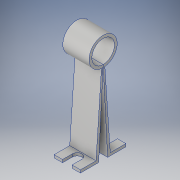
# Autodesk Inventor part: baringstand
Saved by Autodesk Inventor 2018 (Build 220112000, 112)
## iProperties
Created: 2018-02-15
Part Number: baringstand
Material: Aluminum 6061
Document SubType Name: Modeling
Designer: 238438
Density: 2.7 g/cm^3
Appearance: Aluminum - Flat
Author: 238438
Autodesk Inventor part; units mm, degrees
ref_plane "YZ Plane" through (0, 0, 0) normal (1, 0, 0) x (0, 1, 0)
ref_plane "XZ Plane" through (0, 0, 0) normal (0, 1, 0) x (-1, 0, 0)
ref_plane "XY Plane" through (0, 0, 0) normal (0, 0, 1) x (1, 0, 0)
sketch "Sketch2" plane through (0, 0, 0) normal (1, 0, 0) x (0, 1, 0)
  arc A0 (-4.8535, -0.5919) -> (-4.8535, 0.5919) centre (0, 0) ccw
  circle A1 centre (0, 0) radius 3.937
  line L0 (-32.6965, -1.5621) -> (-32.6965, -4.1021)
  line L1 (-31.7186, 2.4716) -> (-4.8535, 0.5919)
  line L2 (-31.7186, -2.4716) -> (-4.8535, -0.5919)
  line L3 (-32.6965, 1.5621) -> (-4.7217, 0.0432)
  line L4 (-32.6965, -1.5621) -> (-4.7217, -0.0423)
  line L5 (-4.7217, 0.0432) -> (-3.937, 0.0003)
  line L6 (-4.7217, -0.0423) -> (-3.937, 0.0003)
  line L7 (-31.7186, -2.4716) -> (-31.7186, -7.9121)
  line L8 (-31.7186, -7.9121) -> (-32.6965, -7.9121)
  line L9 (-32.6965, -7.9121) -> (-32.6965, -1.5621)
  line L10 (-31.7186, 2.4716) -> (-31.7186, 7.9121)
  line L11 (-31.7186, 7.9121) -> (-32.6965, 7.9121)
  line L12 (-32.6965, 7.9121) -> (-32.6965, 1.5621)
  point P0 (-4.7217, 0.5827)
  point P1 (-4.7217, -0.5827)
  point P2 (-32.6965, 0.9779)
  point P3 (-32.6965, 0)
  dimension "d3" = 7.874
  dimension "d2" = 9.779
  constraints: 26 end point, 6 coincident, 2 parallel, 2 point on circle, 2 point on line, 1 centre point, 1 collinear, 3 other
  measures "d2" diameter of A0
extrude "Extrusion1" add sketch "Sketch2" along normal blind 9.144
sketch "Sketch3" plane through (0, -32.6965, 1.5621) normal (0, -1, 0) x (1, 0, 0)
  line L0 (0, 6.35) -> (9.144, 6.35) projected
  line L1 (9.144, 6.35) -> (9.144, 0) projected
  line L2 (2.921, 6.35) -> (2.921, 2.921)
  line L3 (6.223, 2.921) -> (6.223, 6.35)
  arc A0 (2.921, 2.921) -> (6.223, 2.921) centre (4.572, 2.921) ccw
  line L4 (-1.4009, -1.5621) -> (13.744, -1.5621)
  line L5 (2.921, -9.4742) -> (2.921, -6.0452)
  line L6 (6.223, -6.0452) -> (6.223, -9.4742)
  arc A1 (6.223, -6.0452) -> (2.921, -6.0452) centre (4.572, -6.0452) ccw
  line L7 (2.921, -9.4742) -> (6.223, -9.4742)
  line L8 (0, -9.4742) -> (9.144, -9.4742) projected
  point P0 (0, -1.5621)
  dimension "d14" = 2.921
  dimension "d15" = 2.921
  constraints: 12 end point, 5 symmetric about line, 4 point on circle, 2 centre point, 2 point on line, 1 collinear, 1 horizontal, 1 tangent, 1 vertical, 1 other
  measures "d14" distance from line of L1 L3.end
  measures "d15" distance of L0.start L2.start
extrude "Extrusion2" cut sketch "Sketch3" against normal blind 9.144
body "Solid1"
